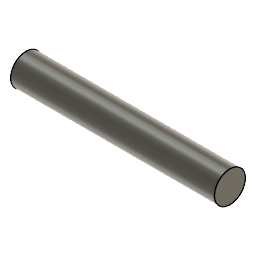
LegPadsPivot (Autodesk Fusion 360 design; units mm, degrees)
part number: 2026-06-01-03-24-19-340
Autodesk Fusion 360 part; units mm, degrees
sketch "PivotSection" plane through (0, 0, 0) normal (1, 0, 0) x (0, 1, 0)
  circle A0 centre (0, 0) radius 4.9
  dimension "d1" = 9.8
  constraint coincident A0.centre origin
  measures "d1" diameter of A0
extrude "Extrude1" add sketch "PivotSection" along normal blind 64.2
named bodies: "LegPadsPivot"
